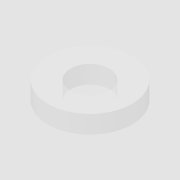
# Autodesk Inventor part: Washer, Teflon, 0.08''
Saved by Autodesk Inventor 2018 (Build 220112000, 112)
## iProperties
Category: Motion
Company: Super Sonic Sparks, Team 24
Part Number: Washer, Teflon, 0.08''
Document SubType Name: Modeling
Designer: Jordan Kiesel
Density: 2.02 g/cm^3
Material: Polytetrafluoroethylene
Mass: 0.120871 g
Surface Area: 1.5883 cm^2
Volume: 0.0598373 cm^3
Catalog Web Link: vexrobotics.com/washers.html
Description: Use on shafts where metal rubs on metal.
Vendor: VEX Robotics, Inc.
Appearance: Clear
Created: 2017-10-17
Translation Standard: STEP AP203
FileName: Washer, Teflon, 0.04''.ipt
PreProcessor: SolidWorks 2006052
PostProcessor: Build: 239, Release: 2011 RTM - Date: Wed 02/17/2010
Sent Units: inch
Uncertainty: 1e-05
Author: Jordan Kiesel
Title: Washer, Teflon, 0.04"
Comments: A washer is a thin disk with a hole used to distribute the load of a threaded fastener. VEX washers fit on all VEX screws and VEX shafts. ▷ Telfon has low friction. Use on shafts where metal rubs on metal.
Autodesk Inventor part; units mm, degrees
ref_plane "YZ Plane" through (0, 0, 0) normal (1, 0, 0) x (0, 1, 0)
ref_plane "XZ Plane" through (0, 0, 0) normal (0, 1, 0) x (-1, 0, 0)
ref_plane "XY Plane" through (0, 0, 0) normal (0, 0, 1) x (1, 0, 0)
ref_plane "Work Plane3" through (0, 1.0668, 0) normal (0, 1, 0) x (1, 0, 0)
sketch "Sketch1" plane through (0, 1.0668, 0) normal (0, 1, 0) x (1, 0, 0)
  circle A0 centre (0, 0) radius 4.7625
  circle A1 centre (0, 0) radius 2.1971 projected
  circle A2 centre (0, 0) radius 2.1971
  constraints: 2 centre point, 2 coincident
extrude "Extrusion1" add sketch "Sketch1" along normal blind 2.032
body "Solid2"
